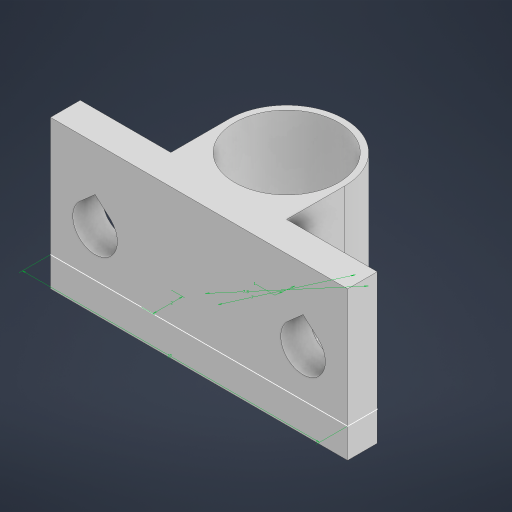
# Autodesk Inventor part: w
Saved by Autodesk Inventor 2024.2 (Build 282272000, 272)
## iProperties
Created: 2024-10-16
Part Number: w
Material: Generic
Document SubType Name: Modeling
Designer: jerem
Density: 1 g/cm^3
Appearance: Default
Author: jerem
## iProperties of the stored document w_3DPrint.ipt
Created: 2024-10-16
Part Number: w_3DPrint
Material: Generic
Document SubType Name: Modeling
Designer: jerem
Density: 1 g/cm^3
Appearance: Default
Author: jerem
Autodesk Inventor part; units mm, degrees
ref_plane "YZ Plane" through (0, 0, 0) normal (1, 0, 0) x (0, 1, 0)
ref_plane "XZ Plane" through (0, 0, 0) normal (0, 1, 0) x (-1, 0, 0)
ref_plane "XY Plane" through (0, 0, 0) normal (0, 0, 1) x (1, 0, 0)
sketch "Sketch1" plane through (0, 0, 0) normal (0, 1, 0) x (-1, 0, 0)
  circle A0 centre (0, 0) radius 3.5
  circle A1 centre (0, 0) radius 3.9
  circle A2 centre (0, 0) radius 0.5
  line L0 (3.9, 0) -> (3.9, 3.9)
  line L1 (3.9, 3.9) -> (0, 3.9)
  line L2 (-3.9, 0) -> (-3.9, 3.9)
  line L3 (-3.9, 3.9) -> (0, 3.9)
  line L4 (3.9, 3.9) -> (3.9, 5.9)
  line L5 (3.9, 5.9) -> (-3.9, 5.9)
  line L6 (-3.9, 5.9) -> (-3.9, 3.9)
  line L7 (3.9, 5.9) -> (10, 5.9)
  line L8 (10, 5.9) -> (10, 3.9)
  line L9 (10, 3.9) -> (3.9, 3.9)
  line L10 (-3.9, 5.9) -> (-10, 5.9)
  line L11 (-10, 5.9) -> (-10, 3.9)
  line L12 (-10, 3.9) -> (-3.9, 3.9)
  dimension "d0" = 7
  dimension "d1" = 7.8
  dimension "d2" = 1
  dimension "d7" = 2
  dimension "d10" = 20
  constraints: 26 end point, 8 perpendicular, 3 centre point, 3 coincident, 3 point on circle, 3 tangent, 2 horizontal, 2 point on line, 2 vertical, 1 collinear
  measures "d0" diameter of A0
  measures "d1" diameter of A1
  measures "d2" diameter of A2
  measures "d7" distance between parallel lines of L1 L5
  measures "d10" distance between parallel lines of L11 L8
extrude "Extrusion1" add sketch "Sketch1" along normal blind 8 contours A1 | A1 L1 L0 | L3 L6 L5 L4 L1 | A1 L2 L3 | L4 L7 L8 L9 | L12 L11 L10 L6
extrude "Extrusion2" add sketch "Sketch1" against normal blind 2 contours A0 | A1 | A1 L1 L0 | L3 L6 L5 L4 L1 | A1 L2 L3 | L4 L7 L8 L9 | L12 L11 L10 L6
sketch "Sketch2" plane through (10, 8, 3.9) normal (0, 0, -1) x (-1, 0, 0)
  circle A0 centre (3, -5) radius 1.5
  circle A1 centre (17, -5) radius 1.5
  line L0 (3, -5) -> (17, -5) construction
  line L1 (0, -10) -> (0, 0) construction
  line L2 (20, -10) -> (20, 0) construction
  line L3 (0, 0) -> (6.1, 0) projected
  line L4 (3, -3.5) -> (3, -3) construction
  line L5 (3, -3) -> (3.9922, -3.875)
  line L6 (3, -3) -> (2.0078, -3.875)
  line L7 (17, -3.5) -> (17, -3) construction
  line L8 (17, -3) -> (16.0078, -3.875)
  line L9 (17, -3) -> (17.9922, -3.875)
  point P0 (10, -8)
  dimension "d11" = 3
  dimension "d12" = 3
  dimension "d13" = 3
  dimension "d14" = 3
  dimension "d15" = 5
  dimension "d18" = 0.5
  dimension "d19" = 0.5
  constraints: 14 end point, 6 point on circle, 4 tangent, 2 centre point, 2 line through centre, 2 vertical, 1 horizontal
  measures "d11" distance from line of L1 L0.start
  measures "d12" diameter of A0
  measures "d13" diameter of A1
  measures "d14" distance from line of L2 L0.end
  measures "d15" distance from line of L0.start L3
  measures "d18" distance of L4.start L4.end
  measures "d19" distance of L7.start L7.end
extrude "Extrusion3" cut sketch "Sketch2" against normal through all
equation "\"d13\" = d12"
equation "\"d14\" = d11"
equation "\"d19\" = d18"
body "Solid1"
